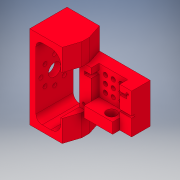
# Autodesk Inventor part: EDMO1-0_Body
Saved by Autodesk Inventor 2019 (Build 230136000, 136)
## iProperties
Created: 2016-10-24
Part Number: EDMO1-0_Body
Material: PLA
Document SubType Name: Modeling
Designer: Lucas
Density: 1.29985 g/cm^3
Appearance: Default
Mass: 47.5353 g
Surface Area: 164.605 cm^2
Volume: 36.5698 cm^3
Author: Lucas
Autodesk Inventor part; units mm, degrees
ref_plane "YZ Plane" through (0, 0, 0) normal (1, 0, 0) x (0, 1, 0)
ref_plane "XZ Plane" through (0, 0, 0) normal (0, 1, 0) x (-1, 0, 0)
ref_plane "XY Plane" through (0, 0, 0) normal (0, 0, 1) x (1, 0, 0)
sketch "Sketch2" plane through (0, 0, 0) normal (0, 0, 1) x (1, 0, 0)
  line L0 (0, 0) -> (42, 0)
  line L1 (42, 0) -> (42, 32)
  line L2 (42, 32) -> (0, 32)
  line L3 (0, 32) -> (0, 0)
  dimension "d0" = 42
  dimension "d1" = 32
  constraints: 8 end point, 2 parallel, 1 horizontal, 1 perpendicular
  measures "d0" distance of L2.end L1.end
  measures "d1" distance of L1.end L0.end
extrude "Body_body" add sketch "Sketch2" along normal blind 15
sketch "Sketch4" plane through (0, 0, 15) normal (0, 0, 1) x (1, 0, 0)
  line L0 (42, 32) -> (0, 32) projected
  line L1 (0, 32) -> (0, 0) projected
  line L2 (4, 24.6) -> (9.5, 24.6)
  line L3 (9.5, 24.6) -> (9.5, 8.6)
  line L4 (9.5, 8.6) -> (32.5, 8.6)
  line L5 (32.5, 8.6) -> (32.5, 24.6)
  line L6 (32.5, 24.6) -> (38, 24.6)
  line L7 (42, 0) -> (42, 32) projected
  line L8 (0, 0) -> (42, 0) projected
  line L9 (4, 24.6) -> (4, 27.1)
  line L10 (4, 27.1) -> (9.5, 27.1)
  line L11 (9.5, 27.1) -> (9.5, 32)
  line L12 (38, 27.1) -> (38, 24.6)
  line L13 (38, 27.1) -> (32.5, 27.1)
  line L14 (32.5, 27.1) -> (32.5, 32)
  line L15 (9.5, 32) -> (32.5, 32)
  line L16 (21, 36.5125) -> (21, -47.625) construction
  point P0 (4.9935, 32)
  point P1 (37, 32)
  dimension "d6" = 5.5
  dimension "d7" = 16
  dimension "d8" = 23
  dimension "d11" = 8.6
  dimension "d14" = 2.5
  dimension "d15" = 2.5
  dimension "d22" = 42
  dimension "d23" = 21
  dimension "d24" = 23
  dimension "d25" = 11.5
  dimension "d26" = 4.9
  dimension "d27" = 4.9
  dimension "d28" = 5.5
  constraints: 26 end point, 6 perpendicular, 4 horizontal, 4 point on line, 3 collinear, 2 vertical
  measures "d6" distance of L2.start L2.end
  measures "d7" distance of L2.end L3.end
  measures "d8" distance of L3.end L4.end
  measures "d11" distance between parallel lines of L8 L4
  measures "d14" distance of L2.start L9.end
  measures "d15" distance of L12.start L6.end
  measures "d22" distance between parallel lines of L7 L1
  measures "d23" distance between parallel lines of L16 L1
  measures "d24" distance between parallel lines of L14 L11
  measures "d25" distance between parallel lines of L16 L11
  measures "d26" distance of L10.end L11.end
  measures "d27" distance of L13.end L14.end
  measures "d28" distance of L12.start L13.end
extrude "Servo_Intake" cut sketch "Sketch4" against normal blind 6.25 contours L14 L13 L12 L6 L5 L4 L3 L2 L9 L10 L11 L0
sketch "Sketch5" plane through (0, 0, 15) normal (0, 0, 1) x (1, 0, 0)
  line L0 (42, 0) -> (42, 32) projected
  line L1 (42, 14.6) -> (42, 13.1)
  line L2 (-29.647, 13.85) -> (54.8226, 13.85) construction
  line L3 (0, 0) -> (42, 0) projected
  line L4 (32.5, 8.6) -> (9.5, 8.6) projected
  line L5 (42, 13.1) -> (32.5, 13.1)
  line L6 (32.5, 13.1) -> (32.5, 14.6)
  line L7 (32.5, 24.6) -> (32.5, 8.6) projected
  line L8 (42, 14.6) -> (32.5, 14.6)
  dimension "d171" = 1.5
  dimension "d211" = 4.5
  constraints: 10 end point, 2 point on line, 1 horizontal, 1 perpendicular, 1 other
  measures "d171" distance between parallel lines of L8 L5
  measures "d211" distance between parallel lines of L5 L4
extrude "Cable_Opening" cut sketch "Sketch5" against normal blind 2.5
sketch "Sketch6" plane through (0, 0, 15) normal (0, 0, 1) x (1, 0, 0)
  circle A0 centre (3.5, 28) radius 1.1 construction
  circle A1 centre (38.5, 28) radius 1.1
  circle A2 centre (38.5, 4) radius 1.1 construction
  circle A3 centre (3.5, 4) radius 1.1
  line L0 (21, 34.35) -> (21, -13.275) construction
  line L1 (-20.6375, 16) -> (66.675, 16) construction
  line L2 (42, 14.6) -> (42, 32) projected
  line L3 (0, 32) -> (0, 0) projected
  line L4 (9.5, 32) -> (0, 32) projected
  line L5 (0, 0) -> (42, 0) projected
  point P0 (42, 12.35)
  point P1 (0, 12.35)
  dimension "d29" = 2.2
  dimension "d30" = 2.2
  dimension "d31" = 2.2
  dimension "d32" = 2.2
  dimension "d33" = 42
  dimension "d34" = 21
  dimension "d35" = 32
  dimension "d36" = 16
  dimension "d37" = 35
  dimension "d38" = 17.5
  dimension "d39" = 24
  dimension "d40" = 12
  constraints: 4 centre point, 4 end point, 2 horizontal alignment, 2 vertical alignment, 1 horizontal
  measures "d29" diameter of A0
  measures "d30" diameter of A1
  measures "d31" diameter of A2
  measures "d32" diameter of A3
  measures "d33" distance between parallel lines of L2 L3
  measures "d34" distance between parallel lines of L0 L3
  measures "d35" distance between parallel lines of L4 L5
  measures "d36" distance between parallel lines of L4 L1
  measures "d37" distance of A1.centre A0.centre
  measures "d38" distance from line of L0 A0.centre
  measures "d39" distance of A3.centre A0.centre
  measures "d40" distance from line of L1 A2.centre
extrude "Holes_Mounting_Screws" cut sketch "Sketch6" against normal up to surface (15 mm away)
sketch "Sketch10" plane through (0, 0, 15) normal (0, 0, 1) x (1, 0, 0)
  line L0 (32.5, 8.6) -> (9.5, 8.6) projected
  line L1 (9.5, 8.6) -> (32.5, 8.6)
  line L2 (32.5, 8.6) -> (32.5, 0)
  line L3 (32.5, 0) -> (9.5, 0)
  line L4 (9.5, 0) -> (9.5, 8.6)
  line L5 (9.5, 8.6) -> (9.5, 24.6) projected
  line L6 (32.5, 24.6) -> (32.5, 14.6) projected
  point P0 (0, 0)
  point P1 (9.5, 12.35)
  point P2 (32.5, 12.35)
  constraints: 8 end point, 2 collinear, 2 parallel, 1 horizontal, 1 perpendicular
extrude "Socket" add sketch "Sketch10" along normal blind 5.8
sketch "Sketch11" plane through (9.5, 8.6, 8.75) normal (0, 1, 0) x (1, 0, 0)
  circle A0 centre (16.25, -6.25) radius 1.6
  line L0 (-9.5, -6.05) -> (-9.5, -3.55) projected
  line L1 (32.5, 8.75) -> (32.5, -6.25) projected
  point P0 (-9.5, 8.75)
  point P1 (0, -6.25)
  dimension "d65" = 3.2
  dimension "d69" = 16.25
  constraints: 1 centre point, 1 horizontal alignment
  measures "d65" diameter of A0
  measures "d69" distance from line of L1 A0.centre
extrude "Shaft_Opening" cut sketch "Sketch11" against normal up to surface (8.6 mm away)
sketch "Sketch12" plane through (9.5, 8.6, 8.75) normal (0, 1, 0) x (1, 0, 0)
  circle A0 centre (16.25, -6.25) radius 4
  circle A1 centre (16.25, -6.25) radius 1.6 projected
  point P0 (-9.5, 8.75)
  dimension "d73" = 8
  constraints: 1 centre point, 1 concentric
  measures "d73" diameter of A0
extrude "Shaft_Pocket" cut sketch "Sketch12" against normal blind 5.7
sketch "Sketch15" plane through (0, 0, 15) normal (0, 0, 1) x (1, 0, 0)
  line L0 (9.5, 32) -> (0, 32) projected
  line L1 (0, 0) -> (9.5, 0) projected
  line L2 (42, 32) -> (32.5, 32) projected
  line L3 (32.5, 0) -> (42, 0) projected
  line L4 (42, 32) -> (0, 32) projected
  line L5 (0, 32) -> (0, 44.5)
  line L6 (0, 44.5) -> (-20, 44.5)
  line L7 (0, 32) -> (5, 32)
  line L8 (5, 32) -> (5, 49.5)
  line L9 (5, 49.5) -> (-25, 49.5)
  line L10 (0, 0) -> (0, -12.5)
  line L11 (0, -12.5) -> (-20, -12.5)
  line L12 (-20, -12.5) -> (-20, 44.5)
  line L13 (0, 0) -> (5, 0)
  line L14 (5, 0) -> (5, -17.5)
  line L15 (5, -17.5) -> (-25, -17.5)
  line L16 (-25, -17.5) -> (-25, 49.5)
  line L17 (0, 32) -> (0, 0) projected
  dimension "d111" = 12.5
  dimension "d113" = 5
  dimension "d114" = 17.5
  dimension "d116" = 12.5
  dimension "d118" = 5
  dimension "d119" = 17.5
  dimension "d120" = 30
  dimension "d161" = 5
  dimension "d175" = 30
  dimension "d191" = 5
  dimension "d212" = 25
  constraints: 24 end point, 7 perpendicular, 2 parallel, 2 point on line, 1 collinear, 1 vertical
  measures "d111" distance of L0.end L5.end
  measures "d113" distance of L0.end L7.end
  measures "d114" distance of L7.end L8.end
  measures "d116" distance of L1.start L10.end
  measures "d118" distance of L1.start L13.end
  measures "d119" distance of L13.end L14.end
  measures "d120" distance of L14.end L15.end
  measures "d161" distance between parallel lines of L15 L11
  measures "d175" distance of L8.end L9.end
  measures "d191" distance between parallel lines of L16 L12
  measures "d212" distance between parallel lines of L17 L16
extrude "Connection_Adapter" add sketch "Sketch15" along normal mid plane 30 contours L0 L5 L6 L12 L11 L10 L1 L14 L15 L16 L9 L8
sketch "Sketch17" plane through (-20, -12.5, 30) normal (1, 0, 0) x (0, 0, -1)
  circle A0 centre (15, 28.5) radius 11 construction
  line L0 (30, 57) -> (0, 57) projected
  line L1 (30, 0) -> (0, 0) projected
  line L2 (0, 0) -> (0, 57) projected
  line L3 (30, 57) -> (30, 0) projected
  line L4 (15, 15.142) -> (15, 40.542) construction
  line L5 (1.1452, 28.5) -> (27.1241, 28.5) construction
  line L6 (4.9901, 18.4901) -> (35.9566, 49.4566) construction
  line L7 (5.2574, 38.2426) -> (22.7782, 20.7218) construction
  circle A1 centre (7.2218, 20.7218) radius 1.65
  circle A2 centre (4, 28.5) radius 1.65
  circle A3 centre (7.2218, 36.2782) radius 1.65
  circle A4 centre (15, 39.5) radius 1.65
  circle A5 centre (15, 17.5) radius 1.65
  circle A6 centre (22.7782, 20.7218) radius 1.65
  circle A7 centre (26, 28.5) radius 1.65
  circle A8 centre (22.7782, 36.2782) radius 1.65
  point P0 (30, 12.5)
  dimension "d121" = 22
  dimension "d122" = 57
  dimension "d123" = 28.5
  dimension "d124" = 30
  dimension "d125" = 15
  dimension "d126" = 3.3
  dimension "d127" = 3.3
  dimension "d128" = 3.3
  dimension "d129" = 3.3
  dimension "d130" = 3.3
  dimension "d131" = 3.3
  dimension "d132" = 3.3
  dimension "d133" = 3.3
  dimension "d134" = 45
  dimension "d135" = 45
  constraints: 11 point on line, 8 centre point, 8 end point, 1 coincident, 1 horizontal, 1 vertical, 10 other
  measures "d122" distance between parallel lines of L0 L1
  measures "d123" distance from line of point (15, 28.5) L1
  measures "d124" distance between parallel lines of L2 L3
  measures "d125" distance from line of L2 point (15, 28.5)
  measures "d126" diameter of A1
  measures "d127" diameter of A2
  measures "d128" diameter of A3
  measures "d129" diameter of A4
  measures "d130" diameter of A5
  measures "d131" diameter of A6
  measures "d132" diameter of A7
  measures "d133" diameter of A8
  measures "d134" angle of L6 L4
  measures "d135" angle of L4 L7
extrude "Connector_Holes" cut sketch "Sketch17" against normal up to surface (5 mm away) contours A1 | A2 | A3 | A4 | A5 | A6 | A7 | A8
sketch "Sketch19" plane through (-20, -12.5, 30) normal (1, 0, 0) x (0, 0, -1)
  circle A0 centre (15, 28.5) radius 5
  line L0 (30, 0) -> (0, 0) projected
  line L1 (30, 57) -> (0, 57) projected
  line L2 (30, 57) -> (30, 0) projected
  line L3 (0, 0) -> (0, 57) projected
  point P0 (30, 12.5)
  dimension "d140" = 10
  dimension "d141" = 57
  dimension "d142" = 28.5
  dimension "d143" = 30
  dimension "d144" = 15
  constraints: 1 centre point
  measures "d140" diameter of A0
  measures "d141" distance between parallel lines of L0 L1
  measures "d142" distance from line of L1 A0.centre
  measures "d143" distance between parallel lines of L2 L3
  measures "d144" distance from line of L3 A0.centre
extrude "Connector_Center_Hole" cut sketch "Sketch19" against normal up to surface (5 mm away) contours A0
sketch "Sketch22" plane through (0, 0, 0) normal (0, 0, -1) x (-1, 0, 0)
  circle A0 centre (-38.5, 28) radius 1.1 projected
  line L0 (-3.5, 36.8375) -> (-3.5, -9.2) construction
  line L1 (-42, 0) -> (-42, 32) projected
  line L2 (0, -12.5) -> (0, 44.5) projected
  line L3 (-5, 0) -> (-42, 0) projected
  line L4 (-42, 32) -> (-5, 32) projected
  circle A1 centre (-3.5, 4) radius 1.75
  circle A2 centre (-38.5, 28) radius 1.75
  circle A3 centre (-3.5, 4) radius 1.1 projected
  circle A4 centre (-38.5, 28) radius 1.1 projected
  point P0 (0, 0)
  point P1 (0, -1)
  dimension "d167" = 3.5
  dimension "d168" = 3.5
  dimension "d176" = 2.25
  dimension "d177" = 1.75
  constraints: 4 coincident, 2 centre point, 2 concentric, 2 end point, 1 point on line, 1 vertical
  measures "d167" diameter of A1
  measures "d168" diameter of A2
  measures "d176" distance edge to line of A2 L4
  measures "d177" distance edge to line of A2 L1
extrude "Pocket_Inserts" cut sketch "Sketch22" against normal blind 5
fillet "Fillet4" radius 8 2 edges at (0, 44.5, 15) (0, -12.5, 15)
chamfer "Chamfer1" distance 12 angle 18 1 edges at (5, -8.75, 30) measured on face at (5, -11.6667, 15)
chamfer "Chamfer2" distance 12 angle 18 1 edges at (5, -8.75, 0) measured on face at (5, -11.6667, 11)
chamfer "Chamfer3" distance 12 angle 18 1 edges at (5, 40.75, 30) measured on face at (5, 43.6667, 15)
chamfer "Chamfer4" distance 12 angle 18 1 edges at (5, 40.75, 0) measured on face at (5, 43.6667, 11)
fillet "Fillet5" radius 5 2 edges at (-20, -12.5, 15) (-20, 44.5, 15)
sketch "Sketch24" plane through (0, 0, 8.75) normal (0, 0, 1) x (1, 0, 0)
  circle A0 centre (14.75, 26.6) radius 1.75
  line L0 (9.5, 32) -> (32.5, 32) projected
  line L1 (9.5, 27.1) -> (9.5, 32) projected
  line L2 (32.5, 32) -> (32.5, 27.1) projected
  point P0 (0, 0)
  dimension "d192" = 3.5
  dimension "d193" = 5.4
  dimension "d194" = 5.25
  dimension "d200" = 23
  constraints: 1 centre point
  measures "d192" diameter of A0
  measures "d193" distance from line of L0 A0.centre
  measures "d194" distance from line of L1 A0.centre
  measures "d200" distance between parallel lines of L2 L1
extrude "Heat_dissipation_Hole" cut sketch "Sketch24" against normal up to surface (8.75 mm away)
pattern_linear "Rectangular Pattern1" count 3 spacing 6.25 along (1, 0, 0) count 3 spacing 6.25 along (0, -1, 0) of "Heat_dissipation_Hole"
equation "\"d15\" = d14"
equation "\"d23\" = 0.5 * d22"
equation "\"d25\" = 0.5 * d24"
equation "\"d27\" = d26"
equation "\"d28\" = d6"
equation "\"d34\" = 0.5 * d33"
equation "\"d36\" = 0.5 * d35"
equation "\"d38\" = 0.5 * d37"
equation "\"d40\" = 0.5 * d39"
equation "\"d65\" = d70"
equation "\"d123\" = 0.5 * d122"
equation "\"d125\" = 0.5 * d124"
equation "\"d142\" = 0.5 * d141"
equation "\"d144\" = 0.5 * d143"
equation "\"d167\" = d168"
equation "\"d70\" = 3.2"
body "Solid1"
